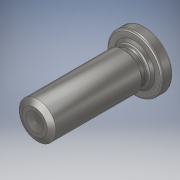
# Autodesk Inventor part: Pin_Headed-2x6mm
Saved by Autodesk Inventor 2018 (Build 220112000, 112)
## iProperties
Created: 2018-07-04
Part Number: Pin_Headed-2x6mm
Material: Stainless Steel
Document SubType Name: Modeling
Designer: Bradley
Density: 8 g/cm^3
Appearance: Semi-Polished
Vendor: 95648A330
Author: Bradley
Autodesk Inventor part; units mm, degrees
ref_plane "YZ Plane" through (0, 0, 0) normal (1, 0, 0) x (0, 1, 0)
ref_plane "XZ Plane" through (0, 0, 0) normal (0, 1, 0) x (-1, 0, 0)
ref_plane "XY Plane" through (0, 0, 0) normal (0, 0, 1) x (1, 0, 0)
sketch "Sketch1" plane through (0, 0, 0) normal (1, 0, 0) x (0, 1, 0)
  line L0 (0.68, 3.039) -> (1, 2.883)
  line L1 (1, 2.883) -> (1, -1.761)
  line L2 (1.12, -2.361) -> (1.41, -2.361)
  line L3 (1.51, -2.461) -> (1.51, -2.861)
  line L4 (1.41, -2.961) -> (0, -2.961)
  line L5 (0, -2.961) -> (0, 2.961)
  arc A0 (1.51, -2.461) -> (1.41, -2.361) centre (1.41, -2.461) ccw
  arc A1 (1.41, -2.961) -> (1.51, -2.861) centre (1.41, -2.861) ccw
  line L6 (0.68, 3.039) -> (0.476, 3.039)
  line L7 (0.476, 3.039) -> (0, 2.961)
  line L8 (1.12, -2.361) -> (1, -2.241)
  arc A2 (1, -1.761) -> (0.85, -1.911) centre (1, -1.911) ccw
  line L9 (0.85, -1.911) -> (0.85, -2.091)
  arc A3 (0.85, -2.091) -> (1, -2.241) centre (1, -2.091) ccw
  point P0 (0, 0)
  point P1 (1.51, -2.361)
  point P2 (1.51, -2.961)
  point P3 (0, 0)
  dimension "d0" = 2
  dimension "d2" = 3.02
  dimension "d4" = 1.36
  dimension "d6" = 0.6
  dimension "d8" = 0.1
  dimension "d9" = 0.156
  dimension "d11" = 6
  dimension "d12" = 0.952
  dimension "d13" = 0.078
  dimension "d14" = 2.24
  dimension "d15" = 135
  dimension "d16" = 0.6
  dimension "d17" = 1.7
  constraints: 20 end point, 8 point on circle, 7 point on line, 6 tangent, 4 centre point, 2 perpendicular, 1 coincident, 1 equal radius, 1 horizontal, 1 midpoint, 1 parallel, 1 vertical, 1 vertical alignment
  measures "d0" diameter of L1 L5
  measures "d2" diameter of L3 L5
  measures "d4" diameter of L0.start L5
  measures "d6" distance of point (1.51, -2.361) point (1.51, -2.961)
  measures "d8" radius of A0
  measures "d9" vertical distance of L0.start L0.end
  measures "d11" distance between parallel lines of L4 L6
  measures "d12" diameter of L6.end L5
  measures "d13" vertical distance of L6.end L5.end
  measures "d14" diameter of L2.start L5
  measures "d15" angle of L2 L8
  measures "d16" distance from line of L1.end L2
  measures "d17" diameter of L9.start L5
revolve "Revolution1" add sketch "Sketch1" angle 360 about axis through (0, 0, -2.961) along (0, 0, 1)
body "Solid1"
